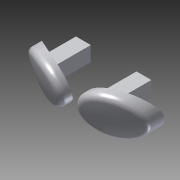
# Autodesk Inventor part: Ojo
Saved by Autodesk Inventor 2014 (Build 180170000, 170)
## iProperties
Created: 2015-01-03
Part Number: Ojo
Material: Generic
Document SubType Name: Modeling
Designer: Rubén
Density: 1 g/cm^3
Appearance: White
d0: 15,000 mm
d1: 2,700 mm
d2: 2,700 mm
d5: 17,000 mm
d6: 20,000 mm
d7: 0,00 deg
d10: 5,500 mm
d11: 2,500 mm
d13: 0,00 deg
d14: 8,000 mm
d15: 0,00 deg
d16: 1,000 mm
Author: Rubén
Autodesk Inventor part; units mm, degrees
ref_plane "YZ Plane" through (0, 0, 0) normal (1, 0, 0) x (0, 1, 0)
ref_plane "XZ Plane" through (0, 0, 0) normal (0, 1, 0) x (-1, 0, 0)
sketch "Sketch2" plane through (0, 0, 0) normal (0, 1, 0) x (-1, 0, 0)
  arc A0 (15, 0) -> (-15, 0) centre (0, 0) ccw
  line L0 (-15, 0) -> (15, 0)
  dimension "d0" = 15
  constraints: 2 end point, 2 point on circle, 1 centre point, 1 coincident, 1 horizontal
  measures "d0" radius of A0
sketch "Sketch3" plane through (0, 0, 0) normal (0, 0, 1) x (1, 0, 0)
  line L0 (-4.15, -1.15) -> (-6.85, -1.15)
  line L1 (-6.85, -1.15) -> (-6.85, -3.85)
  line L2 (-6.85, -3.85) -> (-4.15, -3.85)
  line L3 (-4.15, -3.85) -> (-4.15, -1.15)
  line L4 (0, 0) -> (0, -6.7849) construction
  line L5 (4.15, -1.15) -> (6.85, -1.15)
  line L6 (6.85, -1.15) -> (6.85, -3.85)
  line L7 (6.85, -3.85) -> (4.15, -3.85)
  line L8 (4.15, -3.85) -> (4.15, -1.15)
  line L9 (-6.85, -2.5) -> (-4.15, -2.5) construction
  line L10 (-5.5, -1.15) -> (-5.5, -3.85) construction
  point P0 (-5.5, -2.5)
  dimension "d1" = 2.7
  dimension "d2" = 2.7
  dimension "d10" = 5.5
  dimension "d11" = 2.5
  constraints: 22 end point, 5 midpoint, 4 symmetric about line, 3 parallel, 1 horizontal, 1 perpendicular
  measures "d1" distance of L2.end L1.end
  measures "d2" distance of L1.end L0.end
  measures "d10" horizontal distance of L4.start point (-5.5, -2.5)
  measures "d11" vertical distance of point (-5.5, -2.5) L4.start
sketch "Sketch5" plane through (0, 0, 0) normal (0, 0, 1) x (1, 0, 0)
  ellipse E0 centre (-6, -4) end of major axis (-1.2, -4) minor radius 3.8
  point P0 (0, 0)
  point P1 (-1.2, -4)
  dimension "d19" = 3.8
  dimension "d20" = 4.8
  dimension "d17" = 6
  dimension "d18" = 4
  constraints: 1 coincident, 1 horizontal alignment, 2 other
  measures "d17" horizontal distance of point (-6, -4) point (0, 0)
  measures "d18" vertical distance of point (-6, -4) point (0, 0)
sketch "Sketch6" plane through (0, 0, 0) normal (0, 1, 0) x (-1, 0, 0)
  arc A0 (17, 0) -> (-17, 0) centre (0, 0) ccw
  line L0 (-17, 0) -> (17, 0)
  dimension "d5" = 17
  constraints: 2 end point, 2 point on circle, 1 centre point, 1 coincident, 1 horizontal
  measures "d5" radius of A0
extrude "Extrusion1" add sketch "Sketch5" along normal blind 20
revolve "Revolution1" cut sketch "Sketch2" angle 360 about axis through (15, 0, 0) along (-1, 0, 0)
revolve "Revolution2" cut sketch "Sketch6" angle 360 about axis through (17, 0, 0) along (-1, 0, 0) keep common part
extrude "Extrusion2" add sketch "Sketch3" along normal up to surface contours L3 L2 L1 L0
sketch "Sketch7" plane through (0, 0, 0) normal (0, 0, -1) x (-1, 0, 0)
  line L0 (4.15, -1.15) -> (6.85, -1.15) projected
  line L1 (4.15, -3.85) -> (4.15, -1.15) projected
  line L2 (6.85, -3.85) -> (4.15, -3.85) projected
  line L3 (6.85, -1.15) -> (6.85, -3.85) projected
  point P0 (0, 0)
extrude "Extrusion3" cut sketch "Sketch7" against normal blind 8
fillet "Fillet1" radius 1 1 edges at (-10.7977, -3.882, 12.5435)
ref_plane "Work Plane1" through (0, 0, 0) normal (-1, 0, 0) x (0, -1, 0)
mirror "Mirror1" about plane through (0, 0, 0) normal (-1, 0, 0)
body "Solid1"
